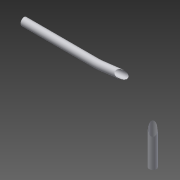
# Autodesk Inventor part: Rura_podłużna_ergosiedziska_lewa
Saved by Autodesk Inventor 2015 (Build 190159000, 159)
## iProperties
Created: 2015-11-20
Part Number: Rura_podłużna_ergosiedziska_lewa
Material: Aluminium AW-7020
Document SubType Name: Modelowanie
Designer: graaapsik
Density: 2.78 g/cm^3
Appearance: Aluminium AW-7020
Sheet Metal Rule: Default
Author: graaapsik
Autodesk Inventor part; units mm, degrees
ref_plane "YZ Plane" through (0, 0, 0) normal (1, 0, 0) x (0, 1, 0)
ref_plane "XZ Plane" through (0, 0, 0) normal (0, 1, 0) x (-1, 0, 0)
ref_plane "XY Plane" through (0, 0, 0) normal (0, 0, 1) x (1, 0, 0)
sketch "Szkic1" plane through (0, 0, 0) normal (1, 0, 0) x (0, 1, 0)
  circle A0 centre (0, 0) radius 16
  dimension "d0" = 32
  constraints: 1 centre point, 1 coincident
  measures "d0" diameter of A0
extrude "Wyciągnięcie proste1" add sketch "Szkic1" along normal blind 815
shell "Skorupa1" thickness 2 removed faces 2 at (815, 4.7224, 2.4785) at (0, 4.7224, 2.4785)
sketch "Szkic4" plane through (0, 0, 0) normal (0, 0, 1) x (1, 0, 0)
  line L0 (320, 29.1092) -> (320, -35.5658)
  line L1 (0, 16) -> (0, -16) projected
  point P0 (0, 0)
  dimension "d8" = 320
  constraints: 2 end point, 1 vertical
  measures "d8" distance between parallel lines of L0 L1
bend part "Gięcie części1" radius 163.7022 angle 7 line through (320, 29.1092, 0) along (0, -1, 0) centre toward (0, 0, 1) moving side (1, 0, 0) both sides no
sketch "Szkic7" plane through (811.4097, 0, 59.1081) normal (0.9925462, 0, 0.1218693) x (0.1218693, 0, -0.9925462)
  circle A0 centre (0, 0) radius 14 projected
  circle A1 centre (0, 0) radius 16 projected
  point P0 (-40.2184, 0)
  point P1 (16, 0)
  constraints: 1 horizontal alignment, 1 other
ref_plane "Płaszczyzna konstrukcyjna4" through (813.3596, 0, 43.2274) normal (0.1218693, 0, -0.9925462) x (0, 1, 0)
sketch "Szkic8" plane through (813.3596, 0, 43.2274) normal (0.1218693, 0, -0.9925462) x (0, 1, 0)
  line L0 (-19.5179, -302.5651) -> (38.9, -302.5651)
  ellipse E0 centre (0, -812.5651) end of major axis (-16, -812.5651) minor radius 1.9499 projected
  dimension "d15" = 510
  constraints: 2 end point, 1 horizontal, 1 other
  measures "d15" distance from line of point (0, -812.565) L0
bend part "Gięcie części2" radius 35.4407 angle 97 line through (513.0498, -19.5179, 6.354) along (0, 1, 0) centre toward (0.1218693, 0, -0.9925462) moving side (0.9925462, 0, 0.1218693) both sides no
sketch "Szkic10" plane through (0, 0, 0) normal (0, 0, 1) x (1, 0, 0)
  line L0 (0, 16) -> (0, -16) construction
  line L1 (0, -16) -> (320, -16) construction
  line L2 (0, 16) -> (0, -16)
  line L3 (0, -16) -> (2.7996, -16)
  line L4 (2.7996, -16) -> (0, 16)
  point P0 (0, 0)
  dimension "d22" = 5
  constraints: 6 end point, 1 perpendicular, 1 point on line
  measures "d22" angle of L4 L2
extrude "Wyciągnięcie proste4" cut sketch "Szkic10" along normal mid plane 32
equation "\"PromieńGięcia\" = Grubość"
equation "\"SzerokośćGięciaPodcięcia\" = Grubość"
equation "\"GłębokośćGięciaPodcięcia\" = 0.5 * Grubość"
equation "\"RozmiarPodcięciaNarożnika\" = 4 * Grubość"
equation "\"MinimalnaPozostałość\" = 2 * Grubość"
equation "\"PromieńPrzejścia\" = PromieńGięcia"
equation "\"Rozmiar_promienia_Jacobiego\" = Grubość"
equation "\"Wielk_odstępu\" = Grubość"
equation "\"Grubość\" = 0.5"
